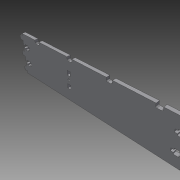
# Autodesk Inventor part: front_panel_bottom
Saved by Autodesk Inventor 2014 (Build 180170000, 170)
## iProperties
Created: 2014-03-23
Part Number: front_panel_bottom
Material: Plywood, Finish
Document SubType Name: Modeling
Designer: buben
Density: 0.552 g/cm^3
Appearance: Plywood - New
Author: buben
Autodesk Inventor part; units mm, degrees
ref_plane "YZ Plane" through (0, 0, 0) normal (1, 0, 0) x (0, 1, 0)
ref_plane "XZ Plane" through (0, 0, 0) normal (0, 1, 0) x (-1, 0, 0)
ref_plane "XY Plane" through (0, 0, 0) normal (0, 0, 1) x (1, 0, 0)
sketch "Sketch1" plane through (0, 0, 0) normal (0, 1, 0) x (-1, 0, 0)
  line L0 (0, 0) -> (-300, 0)
  line L1 (-300, 0) -> (-300, -74.151)
  line L2 (-300, -74.151) -> (0, -74.151)
  line L3 (0, -74.151) -> (0, 0)
  dimension "d0" = 300
  dimension "d1" = 74.151
  constraints: 8 end point, 2 parallel, 1 horizontal, 1 perpendicular
  measures "d0" distance of L0.start L0.end
  measures "d1" distance of L2.end L0.start
extrude "Extrusion1" add sketch "Sketch1" along normal blind 6.5
sketch "Sketch2" plane through (0, 6.5, 0) normal (0, 1, 0) x (1, 0, 0)
  line L0 (0, 0) -> (300, 0) projected
  line L1 (300, 74.151) -> (0, 74.151) projected
  line L2 (150, 74.151) -> (150, 0) construction
  line L3 (34, 0) -> (44, 0)
  line L4 (44, 0) -> (44, 4)
  line L5 (42, 6) -> (36, 6)
  line L6 (34, 4) -> (34, 0)
  line L7 (108, 0) -> (118, 0)
  line L8 (118, 0) -> (118, 4)
  line L9 (116, 6) -> (110, 6)
  line L10 (108, 4) -> (108, 0)
  arc A0 (36, 6) -> (34, 4) centre (36, 4) ccw
  arc A1 (44, 4) -> (42, 6) centre (42, 4) ccw
  arc A2 (110, 6) -> (108, 4) centre (110, 4) ccw
  arc A3 (118, 4) -> (116, 6) centre (116, 4) ccw
  line L11 (266, 0) -> (256, 0)
  line L12 (256, 0) -> (256, 4)
  line L13 (258, 6) -> (264, 6)
  line L14 (266, 4) -> (266, 0)
  line L15 (192, 0) -> (182, 0)
  line L16 (182, 0) -> (182, 4)
  line L17 (184, 6) -> (190, 6)
  line L18 (192, 4) -> (192, 0)
  arc A4 (266, 4) -> (264, 6) centre (264, 4) ccw
  arc A5 (258, 6) -> (256, 4) centre (258, 4) ccw
  arc A6 (192, 4) -> (190, 6) centre (190, 4) ccw
  arc A7 (184, 6) -> (182, 4) centre (184, 4) ccw
  point P0 (39, 6)
  point P1 (113, 6)
  point P2 (261, 6)
  point P3 (187, 6)
  dimension "d10" = 2
  dimension "d11" = 74
  dimension "d12" = 37
  dimension "d13" = 10
  dimension "d14" = 10
  dimension "d15" = 6
  constraints: 34 end point, 18 symmetric about line, 16 point on circle, 8 centre point, 8 tangent, 4 midpoint, 4 parallel, 3 equal radius, 2 horizontal, 2 perpendicular, 2 point on line, 1 collinear, 4 other
  measures "d10" radius of A0
  measures "d11" distance of point (113, 6) point (39, 6)
  measures "d12" distance from line of L2 point (113, 6)
  measures "d13" distance between parallel lines of L6 L4
  measures "d14" distance between parallel lines of L8 L10
  measures "d15" distance between parallel lines of L0 L5
extrude "Extrusion2" cut sketch "Sketch2" against normal through all
sketch "Sketch3" plane through (0, 6.5, 0) normal (0, 1, 0) x (1, 0, 0)
  line L0 (106.75, 53.402) -> (113.25, 53.402)
  line L1 (113.25, 53.402) -> (113.25, 45.402)
  line L2 (113.25, 45.402) -> (106.75, 45.402)
  line L3 (106.75, 45.402) -> (106.75, 53.402)
  line L4 (106.75, 30.402) -> (113.25, 30.402)
  line L5 (113.25, 30.402) -> (113.25, 22.402)
  line L6 (113.25, 22.402) -> (106.75, 22.402)
  line L7 (106.75, 22.402) -> (106.75, 30.402)
  circle A0 centre (110, 37.902) radius 2.25
  line L8 (0, 74.151) -> (0, 0) projected
  line L9 (300, 74.151) -> (0, 74.151) projected
  point P0 (110, 45.402)
  dimension "d18" = 6.5
  dimension "d19" = 8
  dimension "d20" = 15
  dimension "d21" = 4.5
  dimension "d22" = 7.5
  dimension "d56" = 110
  dimension "d57" = 36.249
  constraints: 16 end point, 4 parallel, 3 collinear, 2 horizontal, 2 perpendicular, 1 centre point, 1 midpoint, 1 vertical alignment
  measures "d18" distance of L0.start L0.end
  measures "d19" distance of L2.end L0.start
  measures "d20" distance between parallel lines of L2 L4
  measures "d21" diameter of A0
  measures "d22" distance from line of L2 A0.centre
  measures "d56" distance from line of L8 A0.centre
  measures "d57" distance from line of L9 A0.centre
extrude "Extrusion3" cut sketch "Sketch3" against normal through all
sketch "Sketch4" plane through (0, 6.5, 0) normal (0, 1, 0) x (1, 0, 0)
  line L0 (300, 74.151) -> (0, 74.151) projected
  line L1 (0, 74.151) -> (0, 0) projected
  line L2 (0, 0) -> (34, 0) projected
  line L3 (118, 0) -> (182, 0) projected
  line L4 (0, 70.151) -> (-4.5, 70.151)
  line L5 (-6.5, 68.151) -> (-6.5, 64.151)
  line L6 (-4.5, 62.151) -> (0, 62.151)
  line L7 (0, 62.151) -> (0, 70.151)
  line L8 (0, 41.0755) -> (-4.5, 41.0755)
  line L9 (-6.5, 39.0755) -> (-6.5, 35.0755)
  line L10 (-4.5, 33.0755) -> (0, 33.0755)
  line L11 (0, 33.0755) -> (0, 41.0755)
  line L12 (0, 12) -> (-4.5, 12)
  line L13 (-6.5, 10) -> (-6.5, 6)
  line L14 (-4.5, 4) -> (0, 4)
  line L15 (0, 4) -> (0, 12)
  line L16 (150, 74.151) -> (150, 0) construction
  arc A0 (-4.5, 70.151) -> (-6.5, 68.151) centre (-4.5, 68.151) ccw
  arc A1 (-6.5, 64.151) -> (-4.5, 62.151) centre (-4.5, 64.151) ccw
  arc A2 (-4.5, 41.0755) -> (-6.5, 39.0755) centre (-4.5, 39.0755) ccw
  arc A3 (-6.5, 35.0755) -> (-4.5, 33.0755) centre (-4.5, 35.0755) ccw
  arc A4 (-4.5, 12) -> (-6.5, 10) centre (-4.5, 10) ccw
  arc A5 (-6.5, 6) -> (-4.5, 4) centre (-4.5, 6) ccw
  line L17 (-2.25, 62.151) -> (-2.25, 41.0755) construction
  line L18 (-2.25, 33.0755) -> (-2.25, 12) construction
  line L19 (300, 70.151) -> (304.5, 70.151)
  line L20 (306.5, 68.151) -> (306.5, 64.151)
  line L21 (304.5, 62.151) -> (300, 62.151)
  line L22 (300, 62.151) -> (300, 70.151)
  line L23 (300, 41.0755) -> (304.5, 41.0755)
  line L24 (306.5, 39.0755) -> (306.5, 35.0755)
  line L25 (304.5, 33.0755) -> (300, 33.0755)
  line L26 (300, 33.0755) -> (300, 41.0755)
  line L27 (300, 12) -> (304.5, 12)
  line L28 (306.5, 10) -> (306.5, 6)
  line L29 (304.5, 4) -> (300, 4)
  line L30 (300, 4) -> (300, 12)
  arc A6 (306.5, 68.151) -> (304.5, 70.151) centre (304.5, 68.151) ccw
  arc A7 (304.5, 62.151) -> (306.5, 64.151) centre (304.5, 64.151) ccw
  arc A8 (306.5, 39.0755) -> (304.5, 41.0755) centre (304.5, 39.0755) ccw
  arc A9 (304.5, 33.0755) -> (306.5, 35.0755) centre (304.5, 35.0755) ccw
  arc A10 (306.5, 10) -> (304.5, 12) centre (304.5, 10) ccw
  arc A11 (304.5, 4) -> (306.5, 6) centre (304.5, 6) ccw
  line L31 (302.25, 62.151) -> (302.25, 41.0755) construction
  line L32 (302.25, 33.0755) -> (302.25, 12) construction
  dimension "d35" = 2
  dimension "d36" = 8
  dimension "d37" = 6.5
  dimension "d38" = 4
  dimension "d39" = 8
  dimension "d40" = 8
  dimension "d41" = 4
  constraints: 58 end point, 28 symmetric about line, 24 point on circle, 12 centre point, 12 tangent, 6 midpoint, 6 parallel, 5 equal radius, 3 collinear, 3 horizontal, 3 perpendicular, 3 point on line, 6 other
  measures "d35" radius of A0
  measures "d36" distance between parallel lines of L6 L4
  measures "d37" distance between parallel lines of L1 L5
  measures "d38" distance between parallel lines of L0 L4
  measures "d39" distance between parallel lines of L10 L8
  measures "d40" distance between parallel lines of L14 L12
  measures "d41" distance between parallel lines of L2 L14
extrude "Extrusion4" add sketch "Sketch4" against normal blind 6.5
sketch "Sketch5" plane through (0, 6.5, 0) normal (0, 1, 0) x (1, 0, 0)
  line L0 (300, 74.151) -> (0, 74.151) projected
  line L1 (0, 62.151) -> (0, 41.0755) projected
  line L2 (0, 33.0755) -> (0, 12) projected
  line L3 (118, 0) -> (182, 0) projected
  line L4 (16.3, 53.8633) -> (16.3, 49.3633)
  line L5 (0, 49.3633) -> (0, 53.8632)
  line L6 (5, 56.3633) -> (12.3, 56.3633)
  line L7 (12.3, 46.8633) -> (5, 46.8633)
  line L8 (0, 53.8632) -> (5, 53.8633)
  line L9 (12.3, 53.8633) -> (16.3, 53.8633)
  line L10 (16.3, 49.3633) -> (12.3, 49.3633)
  line L11 (5, 49.3633) -> (0, 49.3633)
  line L12 (5, 46.8633) -> (5, 49.3633)
  line L13 (5, 53.8633) -> (5, 56.3633)
  line L14 (12.3, 56.3633) -> (12.3, 53.8633)
  line L15 (12.3, 49.3633) -> (12.3, 46.8633)
  line L16 (150, 74.151) -> (150, 0) construction
  line L17 (16.3, 24.7878) -> (16.3, 20.2878)
  line L18 (0, 20.2878) -> (0, 24.7877)
  line L19 (5, 27.2877) -> (12.3, 27.2878)
  line L20 (12.3, 17.7878) -> (5, 17.7878)
  line L21 (0, 24.7877) -> (5, 24.7877)
  line L22 (12.3, 24.7878) -> (16.3, 24.7878)
  line L23 (16.3, 20.2878) -> (12.3, 20.2878)
  line L24 (5, 20.2878) -> (0, 20.2878)
  line L25 (5, 17.7878) -> (5, 20.2878)
  line L26 (5, 24.7877) -> (5, 27.2877)
  line L27 (12.3, 27.2878) -> (12.3, 24.7878)
  line L28 (12.3, 20.2878) -> (12.3, 17.7878)
  line L29 (283.7, 53.8633) -> (283.7, 49.3633)
  line L30 (300, 49.3633) -> (300, 53.8633)
  line L31 (295, 56.3633) -> (287.7, 56.3633)
  line L32 (287.7, 46.8633) -> (295, 46.8633)
  line L33 (300, 53.8633) -> (295, 53.8633)
  line L34 (287.7, 53.8633) -> (283.7, 53.8633)
  line L35 (283.7, 49.3633) -> (287.7, 49.3633)
  line L36 (295, 49.3633) -> (300, 49.3633)
  line L37 (295, 46.8633) -> (295, 49.3633)
  line L38 (295, 53.8633) -> (295, 56.3633)
  line L39 (287.7, 56.3633) -> (287.7, 53.8633)
  line L40 (287.7, 49.3633) -> (287.7, 46.8633)
  line L41 (300, 20.2878) -> (300, 24.7878)
  line L42 (300, 24.7878) -> (295, 24.7878)
  line L43 (295, 24.7878) -> (295, 27.2878)
  line L44 (295, 20.2878) -> (300, 20.2878)
  line L45 (295, 17.7878) -> (295, 20.2878)
  line L46 (295, 27.2878) -> (287.7, 27.2878)
  line L47 (287.7, 27.2878) -> (287.7, 24.7878)
  line L48 (287.7, 20.2878) -> (287.7, 17.7878)
  line L49 (287.7, 17.7878) -> (295, 17.7878)
  line L50 (287.7, 24.7878) -> (283.7, 24.7878)
  line L51 (283.7, 20.2878) -> (287.7, 20.2878)
  line L52 (283.7, 24.7878) -> (283.7, 20.2878)
  point P0 (0, 51.6132)
  point P1 (0, 22.5378)
  point P2 (300, 51.6133)
  point P3 (300, 22.5378)
  dimension "d44" = 4.5
  dimension "d45" = 5
  dimension "d46" = 4
  dimension "d47" = 7.3
  dimension "d48" = 2.5
  dimension "d49" = 4.5
  dimension "d50" = 5
  dimension "d51" = 4
  dimension "d52" = 7.3
  dimension "d53" = 2.5
  constraints: 98 end point, 26 symmetric about line, 20 parallel, 10 collinear, 8 perpendicular, 6 horizontal, 6 midpoint
  measures "d44" distance of L4.start L4.end
  measures "d45" distance of L5.end L8.end
  measures "d46" distance of L9.start L4.start
  measures "d47" distance of L6.start L6.end
  measures "d48" distance of L6.end L9.start
  measures "d49" distance of L22.end L23.start
  measures "d50" distance of L18.end L21.end
  measures "d51" distance of L27.end L22.end
  measures "d52" distance of L26.end L19.end
  measures "d53" distance of L19.end L27.end
extrude "Extrusion5" cut sketch "Sketch5" against normal through all
equation "\"d12\" = 0.5 * d11"
equation "\"d13\" = d14"
equation "\"d22\" = 0.5 * d20"
equation "\"d39\" = d36"
equation "\"d40\" = d39"
body "Solid1"
